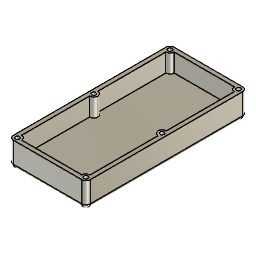
carcasa baqueano (Autodesk Fusion 360 design; units mm, degrees)
Autodesk Fusion 360 part; units mm, degrees
sketch "Boceto1" plane through (0, 0, 0) normal (0, 0, 1) x (1, 0, 0)
  line L0 (-24.5, -57.5) -> (24.5, -57.5)
  line L1 (27.5, -54.5) -> (27.5, 54.5)
  line L2 (24.5, 57.5) -> (-24.5, 57.5)
  line L3 (-27.5, 54.5) -> (-27.5, -54.5)
  arc A0 (-24.5, 57.5) -> (-27.5, 54.5) centre (-24.5, 54.5) ccw
  arc A1 (27.5, 54.5) -> (24.5, 57.5) centre (24.5, 54.5) ccw
  arc A2 (-27.5, -54.5) -> (-24.5, -57.5) centre (-24.5, -54.5) ccw
  arc A3 (24.5, -57.5) -> (27.5, -54.5) centre (24.5, -54.5) ccw
  circle A4 centre (-24.5, 54.5) radius 1.5
  circle A5 centre (24.5, 54.5) radius 1.5
  circle A6 centre (-24.5, -54.5) radius 1.5
  circle A7 centre (24.5, -54.5) radius 1.5
  line L4 (21.5, 54.5) -> (-21.5, 54.5)
  line L5 (-27.5, -57.5) -> (-26.9159, -56.2786) construction
  arc A8 (-27.5, -54.5) -> (-24.5, -57.5) centre (-24.5, -54.5) ccw
  arc A9 (-21.5, -54.5) -> (-24.5, -51.5) centre (-24.5, -54.5) ccw
  line L6 (-21.5, -54.5) -> (21.5, -54.5)
  arc A10 (24.5, -57.5) -> (27.5, -54.5) centre (24.5, -54.5) ccw
  arc A11 (24.5, -51.5) -> (21.5, -54.5) centre (24.5, -54.5) ccw
  line L7 (27.5, -57.5) -> (26.9159, -56.2786) construction
  arc A12 (27.5, 54.5) -> (24.5, 57.5) centre (24.5, 54.5) ccw
  arc A13 (21.5, 54.5) -> (24.5, 51.5) centre (24.5, 54.5) ccw
  arc A14 (-24.5, 57.5) -> (-27.5, 54.5) centre (-24.5, 54.5) ccw
  arc A15 (-24.5, 51.5) -> (-21.5, 54.5) centre (-24.5, 54.5) ccw
  circle A16 centre (-24.5, 0) radius 1.5
  line L8 (-24.5, 51.5) -> (-24.5, 3)
  line L9 (-24.5, -3) -> (-24.5, -51.5)
  arc A17 (-24.5, -3) -> (-24.5, 3) centre (-24.5, 0) ccw
  circle A18 centre (24.5, 0) radius 1.5
  line L10 (24.5, -51.5) -> (24.5, -3)
  line L11 (24.5, 3) -> (24.5, 51.5)
  arc A19 (24.5, 3) -> (24.5, -3) centre (24.5, 0) ccw
  dimension "d3" = 3
  dimension "d4" = 3
  dimension "d5" = 3
  dimension "d6" = 3
  dimension "d7" = 6
  dimension "d8" = 6
  dimension "d9" = 6
  dimension "d10" = 6
  dimension "d11" = 3
  dimension "d12" = 3
  dimension "d13" = 3
  dimension "d14" = 3
  dimension "d15" = 6
  dimension "d16" = 3
  dimension "d17" = 6
  dimension "d18" = 3
  constraint horizontal L0
  constraint perpendicular L0 L1
  constraint parallel L0 L2
  constraint parallel L1 L3
  constraint tangent L2 A0
  constraint tangent L3 A0
  constraint tangent L2 A1
  constraint tangent L1 A1
  constraint coincident L5.start L3
  constraint coincident L5.start L0
  constraint tangent L3 A2
  constraint tangent L0 A2
  constraint coincident L7.start L1
  constraint coincident L7.start L0
  constraint tangent L1 A3
  constraint tangent L0 A3
  constraint concentric A2 A8
  constraint concentric A3 A10
  constraint concentric A0 A14
  constraint concentric A1 A12
  constraint concentric A0 A4
  constraint concentric A1 A5
  constraint concentric A6 A8
  constraint concentric A3 A7
  constraint concentric A8 A9
  constraint concentric A10 A11
  constraint coincident A3 L7.end
  constraint coincident A2 L5.end
  constraint concentric A12 A13
  constraint concentric A14 A15
  constraint concentric A16 A17
  constraint collinear L8 L9
  constraint coincident A16.centre L9
  constraint concentric A18 A19
  constraint collinear L10 L11
  constraint coincident A18.centre L10
  measures "d3" radius of A0
  measures "d4" radius of A1
  measures "d5" radius of A2
  measures "d6" radius of A3
  measures "d7" diameter of A8
  measures "d8" diameter of A10
  measures "d9" diameter of A14
  measures "d10" diameter of A12
  measures "d11" diameter of A4
  measures "d12" diameter of A5
  measures "d13" diameter of A6
  measures "d14" diameter of A7
  measures "d15" diameter of A17
  measures "d16" diameter of A16
  measures "d17" diameter of A19
  measures "d18" diameter of A18
extrude "Extruir1" add sketch "Boceto1" along normal blind 18
extrude "Extruir2" cut sketch "Boceto1" along normal blind 3 contours L0 L1 L2 L3 A0 A1 A2 A3 A8 A10 A12 A14 | A4 | A5 | A6 | A7 | L4 A9 L6 A11 A13 A15 L8 L9 A17 L10 L11 A19 | A16 | A18
extrude "Extruir3" add sketch "Boceto1" along normal blind 3 contours L0 L1 L2 L3 A0 A1 A2 A3 A8 A10 A12 A14 | A4 | A5 | A6 | A7 | L4 A9 L6 A11 A13 A15 L8 L9 A17 L10 L11 A19 | A16 | A18
fillet "Empalme1" radius 3 1 faces at (-9.1667, 18.1667, 0)
extrude "Extruir4" add 1 faces at (-7.4865, 35.5549, 3) along direction (0, 0, 1) blind 2
